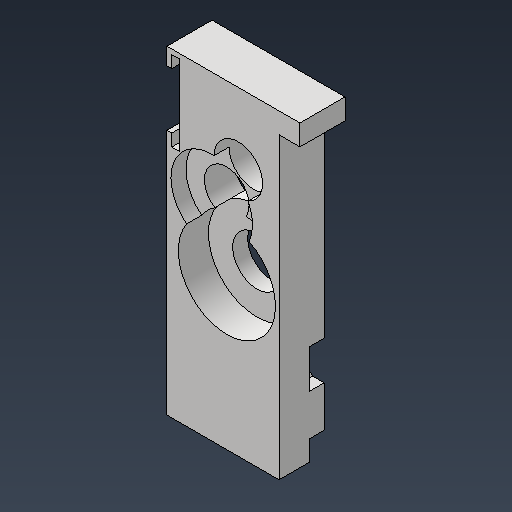
# Autodesk Inventor part: RightGearbox
Saved by Autodesk Inventor 2026.2 (Build 302298010, 298A)
## iProperties
Created: 2026-04-14
Part Number: RightGearbox
Material: Generic
Document SubType Name: Modeling
Designer: szymo
Density: 1 g/cm^3
Appearance: Default
Author: szymo
Autodesk Inventor part; units mm, degrees
ref_plane "YZ Plane" through (0, 0, 0) normal (1, 0, 0) x (0, 1, 0)
ref_plane "XZ Plane" through (0, 0, 0) normal (0, 1, 0) x (-1, 0, 0)
ref_plane "XY Plane" through (0, 0, 0) normal (0, 0, 1) x (1, 0, 0)
sketch "Sketch1" plane through (0, 0, 0) normal (0, 0, 1) x (1, 0, 0)
  circle A0 centre (14.7, -14.7) radius 5
  circle A1 centre (14.7, -14.7) radius 14.7 construction
  circle A2 centre (14.7, -55.6371) radius 5
  circle A3 centre (14.7, -55.6371) radius 14.7 construction
  line L0 (23.1, 0) -> (0, 0)
  line L1 (0, 0) -> (0, -65.8371)
  line L2 (0, -65.8371) -> (23.1, -65.8371)
  line L3 (23.1, -65.8371) -> (23.1, 0)
  circle A4 centre (12.35, -35.2722) radius 5
  line L4 (20.7104, -53.1622) -> (25.128, -48.7446)
  arc A5 (25.128, -48.7446) -> (21.5925, -45.2091) centre (14.7, -55.6371) ccw
  line L5 (21.5925, -45.2091) -> (17.1749, -49.6267)
  arc A6 (20.7104, -53.1622) -> (17.1749, -49.6267) centre (14.7, -55.6371) ccw construction
  arc A7 (4.272, -62.5296) -> (7.8075, -66.0651) centre (14.7, -55.6371) ccw
  line L6 (4.272, -62.5296) -> (8.6896, -58.1119)
  line L7 (12.2251, -61.6475) -> (7.8075, -66.0651)
  line L8 (20.7104, -53.1622) -> (23.1, -53.1622)
  line L9 (21.5925, -45.2091) -> (23.1, -45.2091)
  line L10 (12.2251, -61.6475) -> (8.6896, -58.1119)
  line L11 (20.7104, -53.1622) -> (17.1749, -49.6267)
  line L12 (12.2251, -61.6475) -> (23.1, -61.6475)
  circle A8 centre (9.2226, -23.0665) radius 4.2 construction
  circle A9 centre (9.2226, -23.0665) radius 8 construction
  circle A10 centre (12.35, -35.2722) radius 9.6 construction
  circle A11 centre (12.35, -35.2722) radius 10
  circle A12 centre (9.2226, -23.0665) radius 4.6
  circle A13 centre (9.2226, -23.0665) radius 8.4
  arc A14 (8.6896, -58.1119) -> (12.2251, -61.6475) centre (14.7, -55.6371) ccw construction
  line L13 (2.5, -1) -> (1.5, -1)
  line L14 (1.5, -1) -> (1.5, -17)
  line L15 (1.5, -17) -> (2.5, -17)
  line L16 (2.5, -17) -> (2.5, -1)
  line L17 (1.5, -1) -> (1, -1)
  line L18 (1, -1) -> (1, -3.5)
  line L19 (1, -3.5) -> (0, -3.5)
  line L20 (2.5, -17) -> (2.5, -17.5)
  line L21 (2.5, -17.5) -> (1, -17.5)
  line L22 (1, -17.5) -> (1, -15)
  line L23 (1, -15) -> (0, -15)
  line L24 (23.1, 0) -> (27.4, 0)
  line L25 (27.4, 0) -> (27.4, -4.272)
  line L26 (27.4, -4.272) -> (23.1, -4.272)
  line L27 (7.8075, -4.272) -> (12.2251, -8.6896)
  arc A15 (12.2251, -8.6896) -> (8.6896, -12.2251) centre (14.7, -14.7) ccw
  line L28 (8.6896, -12.2251) -> (4.272, -7.8075)
  arc A16 (7.8075, -4.272) -> (4.272, -7.8075) centre (14.7, -14.7) ccw
  line L29 (7.8075, -4.272) -> (23.1, -4.272)
  circle A17 centre (14.7, -14.7) radius 14.7 construction
  circle A18 centre (14.7, -14.7) radius 14 construction
  circle A19 centre (14.7, -14.7) radius 5 projected
  circle A20 centre (14.7, -14.7) radius 14 construction
  line L30 (10.5645, -8.4432) -> (7.6984, -5.5771) construction
  arc A21 (10.5645, -8.4432) -> (8.4432, -10.5645) centre (14.7, -14.7) ccw construction
  line L31 (5.5771, -7.6984) -> (8.4432, -10.5645) construction
  arc A22 (7.6984, -5.5771) -> (5.5771, -7.6984) centre (14.7, -14.7) ccw construction
  circle A23 centre (14.7, -55.6371) radius 14.7 construction
  circle A24 centre (14.7, -55.6371) radius 14 construction
  line L32 (18.8355, -49.3803) -> (21.7016, -46.5142) projected
  arc A25 (23.8229, -48.6355) -> (21.7016, -46.5142) centre (14.7, -55.6371) ccw projected
  line L33 (23.8229, -48.6355) -> (20.9568, -51.5016) projected
  arc A26 (20.9568, -51.5016) -> (18.8355, -49.3803) centre (14.7, -55.6371) ccw projected
  arc A27 (5.5771, -62.6387) -> (7.6984, -64.76) centre (14.7, -55.6371) ccw projected
  line L34 (5.5771, -62.6387) -> (8.4432, -59.7726) projected
  arc A28 (8.4432, -59.7726) -> (10.5645, -61.8939) centre (14.7, -55.6371) ccw projected
  line L35 (10.5645, -61.8939) -> (7.6984, -64.76) projected
  circle A29 centre (14.7, -55.6371) radius 5 projected
  circle A30 centre (14.7, -55.6371) radius 14 construction
  arc A31 (15.7399, -27.7508) -> (15.8311, -26.3256) centre (9.8372, -26.6574) ccw projected
  arc A32 (15.8311, -26.3256) -> (15.3581, -26.1557) centre (12.35, -35.2722) ccw projected
  arc A33 (15.3581, -26.1557) -> (14.5215, -27.3131) centre (19.7705, -30.2259) ccw projected
  arc A34 (14.5215, -27.3131) -> (14.102, -27.2104) centre (12.35, -35.2722) ccw projected
  arc A35 (14.102, -27.2104) -> (13.8949, -25.7973) centre (8.101, -27.3681) ccw projected
  arc A36 (13.8949, -25.7973) -> (13.3969, -25.7295) centre (12.35, -35.2722) ccw projected
  arc A37 (13.3969, -25.7295) -> (12.8193, -27.0356) centre (18.5592, -28.7934) ccw projected
  arc A38 (12.8193, -27.0356) -> (12.3876, -27.0223) centre (12.35, -35.2722) ccw projected
  arc A39 (12.3876, -27.0223) -> (11.8912, -25.6832) centre (6.5505, -28.4242) ccw projected
  arc A40 (11.8912, -25.6832) -> (11.39, -25.7203) centre (12.35, -35.2722) ccw projected
  arc A41 (11.39, -25.7203) -> (11.0965, -27.118) centre (17.0765, -27.644) ccw projected
  arc A42 (11.0965, -27.118) -> (10.6715, -27.1948) centre (12.35, -35.2722) ccw projected
  arc A43 (10.6715, -27.1948) -> (9.9076, -25.9881) centre (5.2535, -29.7796) ccw projected
  arc A44 (9.9076, -25.9881) -> (9.425, -26.1287) centre (12.35, -35.2722) ccw projected
  arc A45 (9.425, -26.1287) -> (9.4286, -27.5568) centre (15.3872, -26.828) ccw projected
  arc A46 (9.4286, -27.5568) -> (9.0288, -27.7203) centre (12.35, -35.2722) ccw projected
  arc A47 (9.0288, -27.7203) -> (8.0307, -26.6988) centre (4.2666, -31.3751) ccw projected
  arc A48 (8.0307, -26.6988) -> (7.5879, -26.9366) centre (12.35, -35.2722) ccw projected
  arc A49 (7.5879, -26.9366) -> (7.8883, -28.3328) centre (13.5652, -26.3811) ccw projected
  arc A50 (7.8883, -28.3328) -> (7.5312, -28.5758) centre (12.35, -35.2722) ccw projected
  arc A51 (7.5312, -28.5758) -> (6.3426, -27.7842) centre (3.633, -33.1409) ccw projected
  arc A52 (6.3426, -27.7842) -> (5.9589, -28.1088) centre (12.35, -35.2722) ccw projected
  arc A53 (5.9589, -28.1088) -> (6.543, -29.4121) centre (11.6901, -26.3227) ccw projected
  arc A54 (6.543, -29.4121) -> (6.2443, -29.724) centre (12.35, -35.2722) ccw projected
  arc A55 (6.2443, -29.724) -> (4.917, -29.1968) centre (3.3803, -34.9999) ccw projected
  arc A56 (4.917, -29.1968) -> (4.6092, -29.5942) centre (12.35, -35.2722) ccw projected
  arc A57 (4.6092, -29.5942) -> (5.4515, -30.7475) centre (9.8438, -26.6555) ccw projected
  arc A58 (5.4515, -30.7475) -> (5.2242, -31.1147) centre (12.35, -35.2722) ccw projected
  arc A59 (5.2242, -31.1147) -> (3.8163, -30.875) centre (3.5197, -36.8707) ccw projected
  arc A60 (3.8163, -30.875) -> (3.5978, -31.3276) centre (12.35, -35.2722) ccw projected
  arc A61 (3.5978, -31.3276) -> (4.6615, -32.2806) centre (8.107, -27.3648) ccw projected
  arc A62 (4.6615, -32.2806) -> (4.5155, -32.6871) centre (12.35, -35.2722) ccw projected
  arc A63 (4.5155, -32.6871) -> (3.0885, -32.7453) centre (4.045, -38.6717) ccw projected
  arc A64 (3.0885, -32.7453) -> (2.969, -33.2335) centre (12.35, -35.2722) ccw projected
  arc A65 (2.969, -33.2335) -> (4.2075, -33.9445) centre (6.5557, -28.4198) ccw projected
  arc A66 (4.2075, -33.9445) -> (4.1492, -34.3725) centre (12.35, -35.2722) ccw projected
  arc A67 (4.1492, -34.3725) -> (2.7655, -34.7261) centre (4.9333, -40.3241) ccw projected
  arc A68 (2.7655, -34.7261) -> (2.7501, -35.2285) centre (12.35, -35.2722) ccw projected
  arc A69 (2.7501, -35.2285) -> (4.1094, -35.6665) centre (5.2576, -29.7742) ccw projected
  arc A70 (4.1094, -35.6665) -> (4.1414, -36.0972) centre (12.35, -35.2722) ccw projected
  arc A71 (4.1414, -36.0972) -> (2.8615, -36.7308) centre (6.1457, -41.7557) ccw projected
  arc A72 (2.8615, -36.7308) -> (2.9508, -37.2254) centre (12.35, -35.2722) ccw projected
  arc A73 (2.9508, -37.2254) -> (4.3715, -37.3712) centre (4.2695, -31.369) ccw projected
  arc A74 (4.3715, -37.3712) -> (4.4923, -37.7858) centre (12.35, -35.2722) ccw projected
  arc A75 (4.4923, -37.7858) -> (3.3721, -38.6717) centre (7.6293, -42.904) ccw projected
  arc A76 (3.3721, -38.6717) -> (3.5623, -39.1369) centre (12.35, -35.2722) ccw projected
  arc A77 (3.5623, -39.1369) -> (4.9822, -38.9841) centre (3.6346, -33.1343) ccw projected
  arc A78 (4.9822, -38.9841) -> (5.1866, -39.3646) centre (12.35, -35.2722) ccw projected
  arc A79 (5.1866, -39.3646) -> (4.275, -40.464) centre (9.3192, -43.7187) ccw projected
  arc A80 (4.275, -40.464) -> (4.5578, -40.8795) centre (12.35, -35.2722) ccw projected
  arc A81 (4.5578, -40.8795) -> (5.915, -40.4349) centre (3.3805, -34.993) ccw projected
  arc A82 (5.915, -40.4349) -> (6.194, -40.7646) centre (12.35, -35.2722) ccw projected
  arc A83 (6.194, -40.7646) -> (5.5309, -42.0295) centre (11.1416, -44.1643) ccw projected
  arc A84 (5.5309, -42.0295) -> (5.8939, -42.3771) centre (12.35, -35.2722) ccw projected
  arc A85 (5.8939, -42.3771) -> (7.129, -41.66) centre (3.5185, -36.864) ccw projected
  arc A86 (7.129, -41.66) -> (7.4704, -41.9244) centre (12.35, -35.2722) ccw projected
  arc A87 (7.4704, -41.9244) -> (7.0849, -43.2996) centre (13.0167, -44.2212) ccw projected
  arc A88 (7.0849, -43.2996) -> (7.5122, -43.5641) centre (12.35, -35.2722) ccw projected
  arc A89 (7.5122, -43.5641) -> (8.5711, -42.6059) centre (4.0424, -38.6654) ccw projected
  arc A90 (8.5711, -42.6059) -> (8.9601, -42.7936) centre (12.35, -35.2722) ccw projected
  arc A91 (8.9601, -42.7936) -> (8.8689, -44.2188) centre (14.8628, -43.887) ccw projected
  arc A92 (8.8689, -44.2188) -> (9.3419, -44.3887) centre (12.35, -35.2722) ccw projected
  arc A93 (9.3419, -44.3887) -> (10.1785, -43.2313) centre (4.9295, -40.3185) ccw projected
  arc A94 (10.1785, -43.2313) -> (10.598, -43.334) centre (12.35, -35.2722) ccw projected
  arc A95 (10.598, -43.334) -> (10.8051, -44.7471) centre (16.599, -43.1764) ccw projected
  arc A96 (10.8051, -44.7471) -> (11.3031, -44.815) centre (12.35, -35.2722) ccw projected
  arc A97 (11.3031, -44.815) -> (11.8807, -43.5089) centre (6.1408, -41.751) ccw projected
  arc A98 (11.8807, -43.5089) -> (12.3124, -43.5221) centre (12.35, -35.2722) ccw projected
  arc A99 (12.3124, -43.5221) -> (12.8088, -44.8612) centre (18.1495, -42.1202) ccw projected
  arc A100 (12.8088, -44.8612) -> (13.31, -44.8241) centre (12.35, -35.2722) ccw projected
  arc A101 (13.31, -44.8241) -> (13.6035, -43.4264) centre (7.6235, -42.9004) ccw projected
  arc A102 (13.6035, -43.4264) -> (14.0285, -43.3497) centre (12.35, -35.2722) ccw projected
  arc A103 (14.0285, -43.3497) -> (14.7924, -44.5563) centre (19.4465, -40.7648) ccw projected
  arc A104 (14.7924, -44.5563) -> (15.275, -44.4158) centre (12.35, -35.2722) ccw projected
  arc A105 (15.275, -44.4158) -> (15.2714, -42.9876) centre (9.3128, -43.7164) ccw projected
  arc A106 (15.2714, -42.9876) -> (15.6712, -42.8242) centre (12.35, -35.2722) ccw projected
  arc A107 (15.6712, -42.8242) -> (16.6693, -43.8456) centre (20.4334, -39.1693) ccw projected
  arc A108 (16.6693, -43.8456) -> (17.1121, -43.6078) centre (12.35, -35.2722) ccw projected
  arc A109 (17.1121, -43.6078) -> (16.8117, -42.2116) centre (11.1348, -44.1634) ccw projected
  arc A110 (16.8117, -42.2116) -> (17.1688, -41.9686) centre (12.35, -35.2722) ccw projected
  arc A111 (17.1688, -41.9686) -> (18.3574, -42.7603) centre (21.067, -37.4035) ccw projected
  arc A112 (18.3574, -42.7603) -> (18.7411, -42.4356) centre (12.35, -35.2722) ccw projected
  arc A113 (18.7411, -42.4356) -> (18.157, -41.1324) centre (13.0099, -44.2217) ccw projected
  arc A114 (18.157, -41.1324) -> (18.4557, -40.8204) centre (12.35, -35.2722) ccw projected
  arc A115 (18.4557, -40.8204) -> (19.783, -41.3476) centre (21.3197, -35.5446) ccw projected
  arc A116 (19.783, -41.3476) -> (20.0908, -40.9503) centre (12.35, -35.2722) ccw projected
  arc A117 (20.0908, -40.9503) -> (19.2485, -39.7969) centre (14.8562, -43.8889) ccw projected
  arc A118 (19.2485, -39.7969) -> (19.4758, -39.4297) centre (12.35, -35.2722) ccw projected
  arc A119 (19.4758, -39.4297) -> (20.8837, -39.6694) centre (21.1803, -33.6737) ccw projected
  arc A120 (20.8837, -39.6694) -> (21.1022, -39.2168) centre (12.35, -35.2722) ccw projected
  arc A121 (21.1022, -39.2168) -> (20.0385, -38.2638) centre (16.593, -43.1796) ccw projected
  arc A122 (20.0385, -38.2638) -> (20.1845, -37.8573) centre (12.35, -35.2722) ccw projected
  arc A123 (20.1845, -37.8573) -> (21.6115, -37.7991) centre (20.655, -31.8727) ccw projected
  arc A124 (21.6115, -37.7991) -> (21.731, -37.3109) centre (12.35, -35.2722) ccw projected
  arc A125 (21.731, -37.3109) -> (20.4925, -36.5999) centre (18.1443, -42.1246) ccw projected
  arc A126 (20.4925, -36.5999) -> (20.5508, -36.1719) centre (12.35, -35.2722) ccw projected
  arc A127 (20.5508, -36.1719) -> (21.9345, -35.8183) centre (19.7667, -30.2203) ccw projected
  arc A128 (21.9345, -35.8183) -> (21.9499, -35.3159) centre (12.35, -35.2722) ccw projected
  arc A129 (21.9499, -35.3159) -> (20.5906, -34.878) centre (19.4424, -40.7702) ccw projected
  arc A130 (20.5906, -34.878) -> (20.5586, -34.4472) centre (12.35, -35.2722) ccw projected
  arc A131 (20.5586, -34.4472) -> (21.8385, -33.8136) centre (18.5543, -28.7887) ccw projected
  arc A132 (21.8385, -33.8136) -> (21.7492, -33.319) centre (12.35, -35.2722) ccw projected
  arc A133 (21.7492, -33.319) -> (20.3285, -33.1733) centre (20.4305, -39.1755) ccw projected
  arc A134 (20.3285, -33.1733) -> (20.2077, -32.7586) centre (12.35, -35.2722) ccw projected
  arc A135 (20.2077, -32.7586) -> (21.3279, -31.8727) centre (17.0707, -27.6404) ccw projected
  arc A136 (21.3279, -31.8727) -> (21.1377, -31.4075) centre (12.35, -35.2722) ccw projected
  arc A137 (21.1377, -31.4075) -> (19.7178, -31.5603) centre (21.0654, -37.4101) ccw projected
  arc A138 (19.7178, -31.5603) -> (19.5134, -31.1798) centre (12.35, -35.2722) ccw projected
  arc A139 (19.5134, -31.1798) -> (20.425, -30.0804) centre (15.3808, -26.8257) ccw projected
  arc A140 (20.425, -30.0804) -> (20.1422, -29.6649) centre (12.35, -35.2722) ccw projected
  arc A141 (20.1422, -29.6649) -> (18.785, -30.1096) centre (21.3195, -35.5514) ccw projected
  arc A142 (18.785, -30.1096) -> (18.506, -29.7799) centre (12.35, -35.2722) ccw projected
  arc A143 (18.506, -29.7799) -> (19.1691, -28.515) centre (13.5584, -26.3801) ccw projected
  arc A144 (19.1691, -28.515) -> (18.8061, -28.1674) centre (12.35, -35.2722) ccw projected
  arc A145 (18.8061, -28.1674) -> (17.571, -28.8845) centre (21.1815, -33.6804) ccw projected
  arc A146 (17.571, -28.8845) -> (17.2296, -28.62) centre (12.35, -35.2722) ccw projected
  arc A147 (17.2296, -28.62) -> (17.6151, -27.2449) centre (11.6833, -26.3232) ccw projected
  arc A148 (17.6151, -27.2449) -> (17.1878, -26.9803) centre (12.35, -35.2722) ccw projected
  arc A149 (17.1878, -26.9803) -> (16.1289, -27.9385) centre (20.6576, -31.879) ccw projected
  arc A150 (16.1289, -27.9385) -> (15.7399, -27.7508) centre (12.35, -35.2722) ccw projected
  circle A151 centre (9.2226, -23.0665) radius 1.25 projected
  arc A152 (17.1791, -22.2335) -> (16.0134, -21.9938) centre (15.5957, -26.9788) ccw projected
  arc A153 (16.0134, -21.9938) -> (15.948, -21.6398) centre (9.2226, -23.0665) ccw projected
  arc A154 (15.948, -21.6398) -> (16.9509, -20.9991) centre (13.7752, -17.1338) ccw projected
  arc A155 (16.9509, -20.9991) -> (16.8321, -20.5974) centre (9.2226, -23.0665) ccw projected
  arc A156 (16.8321, -20.5974) -> (15.642, -20.6053) centre (16.2699, -25.5683) ccw projected
  arc A157 (15.642, -20.6053) -> (15.5044, -20.2727) centre (9.2226, -23.0665) ccw projected
  arc A158 (15.5044, -20.2727) -> (16.3521, -19.4375) centre (12.4422, -16.3169) ccw projected
  arc A159 (16.3521, -19.4375) -> (16.1524, -19.0693) centre (9.2226, -23.0665) ccw projected
  arc A160 (16.1524, -19.0693) -> (14.99, -19.3244) centre (16.636, -24.0484) ccw projected
  arc A161 (14.99, -19.3244) -> (14.7862, -19.0277) centre (9.2226, -23.0665) ccw projected
  arc A162 (14.7862, -19.0277) -> (15.4418, -18.0345) centre (10.9685, -15.795) ccw projected
  arc A163 (15.4418, -18.0345) -> (15.1699, -17.7159) centre (9.2226, -23.0665) ccw projected
  arc A164 (15.1699, -17.7159) -> (14.0859, -18.2071) centre (16.6782, -22.4856) ccw projected
  arc A165 (14.0859, -18.2071) -> (13.825, -17.9592) centre (9.2226, -23.0665) ccw projected
  arc A166 (13.825, -17.9592) -> (14.2597, -16.8514) centre (9.4186, -15.5909) ccw projected
  arc A167 (14.2597, -16.8514) -> (13.9275, -16.5963) centre (9.2226, -23.0665) ccw projected
  arc A168 (13.9275, -16.5963) -> (12.9693, -17.3022) centre (16.3945, -20.9482) ccw projected
  arc A169 (12.9693, -17.3022) -> (12.6625, -17.114) centre (9.2226, -23.0665) ccw projected
  arc A170 (12.6625, -17.114) -> (12.8574, -15.9399) centre (7.86, -15.7135) ccw projected
  arc A171 (12.8574, -15.9399) -> (12.4795, -15.7595) centre (9.2226, -23.0665) ccw projected
  arc A172 (12.4795, -15.7595) -> (11.689, -16.6491) centre (15.7974, -19.5034) ccw projected
  arc A173 (11.689, -16.6491) -> (11.3498, -16.5288) centre (9.2226, -23.0665) ccw projected
  arc A174 (11.3498, -16.5288) -> (11.2963, -15.3399) centre (6.361, -16.1575) ccw projected
  arc A175 (11.2963, -15.3399) -> (10.8891, -15.242) centre (9.2226, -23.0665) ccw projected
  arc A176 (10.8891, -15.242) -> (10.3009, -16.2766) centre (14.9129, -18.2143) ccw projected
  arc A177 (10.3009, -16.2766) -> (9.944, -16.2295) centre (9.2226, -23.0665) ccw projected
  arc A178 (9.944, -16.2295) -> (9.6445, -15.0776) centre (4.9871, -16.9034) ccw projected
  arc A179 (9.6445, -15.0776) -> (9.2259, -15.0665) centre (9.2226, -23.0665) ccw projected
  arc A180 (9.2259, -15.0665) -> (8.8656, -16.2008) centre (13.7797, -17.1372) ccw projected
  arc A181 (8.8656, -16.2008) -> (8.5068, -16.2289) centre (9.2226, -23.0665) ccw projected
  arc A182 (8.5068, -16.2289) -> (7.9743, -15.1645) centre (3.7983, -17.9187) ccw projected
  arc A183 (7.9743, -15.1645) -> (7.5625, -15.2406) centre (9.2226, -23.0665) ccw projected
  arc A184 (7.5625, -15.2406) -> (7.4459, -16.425) centre (12.4474, -16.3193) ccw projected
  arc A185 (7.4459, -16.425) -> (7.1008, -16.5271) centre (9.2226, -23.0665) ccw projected
  arc A186 (7.1008, -16.5271) -> (6.3587, -15.5967) centre (2.8465, -19.159) ccw projected
  arc A187 (6.3587, -15.5967) -> (5.9717, -15.7568) centre (9.2226, -23.0665) ccw projected
  arc A188 (5.9717, -15.7568) -> (6.1039, -16.9396) centre (10.9741, -15.7963) ccw projected
  arc A189 (6.1039, -16.9396) -> (5.7875, -17.1112) centre (9.2226, -23.0665) ccw projected
  arc A190 (5.7875, -17.1112) -> (4.8682, -16.3554) centre (2.1734, -20.5701) ccw projected
  arc A191 (4.8682, -16.3554) -> (4.523, -16.5925) centre (9.2226, -23.0665) ccw projected
  arc A192 (4.523, -16.5925) -> (4.8982, -17.7219) centre (9.4242, -15.591) ccw projected
  arc A193 (4.8982, -17.7219) -> (4.6244, -17.9555) centre (9.2226, -23.0665) ccw projected
  arc A194 (4.6244, -17.9555) -> (3.5681, -17.4074) centre (1.8085, -22.0902) ccw projected
  arc A195 (3.5681, -17.4074) -> (3.2796, -17.711) centre (9.2226, -23.0665) ccw projected
  arc A196 (3.2796, -17.711) -> (3.8815, -18.7378) centre (7.8656, -15.7125) ccw projected
  arc A197 (3.8815, -18.7378) -> (3.6623, -19.0232) centre (9.2226, -23.0665) ccw projected
  arc A198 (3.6623, -19.0232) -> (2.515, -18.7067) centre (1.7675, -23.653) ccw projected
  arc A199 (2.515, -18.7067) -> (2.296, -19.0637) centre (9.2226, -23.0665) ccw projected
  arc A200 (2.296, -19.0637) -> (3.0982, -19.9428) centre (6.3663, -16.1553) ccw projected
  arc A201 (3.0982, -19.9428) -> (2.9431, -20.2676) centre (9.2226, -23.0665) ccw projected
  arc A202 (2.9431, -20.2676) -> (1.7551, -20.1965) centre (2.0523, -25.1902) ccw projected
  arc A203 (1.7551, -20.1965) -> (1.6152, -20.5913) centre (9.2226, -23.0665) ccw projected
  arc A204 (1.6152, -20.5913) -> (2.5826, -21.2844) centre (4.9918, -16.9002) ccw projected
  arc A205 (2.5826, -21.2844) -> (2.4984, -21.6344) centre (9.2226, -23.0665) ccw projected
  arc A206 (2.4984, -21.6344) -> (1.3216, -21.8118) centre (2.6506, -26.6346) ccw projected
  arc A207 (1.3216, -21.8118) -> (1.2668, -22.227) centre (9.2226, -23.0665) ccw projected
  arc A208 (1.2668, -22.227) -> (2.3572, -22.7039) centre (3.8022, -17.9146) ccw projected
  arc A209 (2.3572, -22.7039) -> (2.3476, -23.0637) centre (9.2226, -23.0665) ccw projected
  arc A210 (2.3476, -23.0637) -> (1.2334, -23.4819) centre (3.536, -27.923) ccw projected
  arc A211 (1.2334, -23.4819) -> (1.2661, -23.8995) centre (9.2226, -23.0665) ccw projected
  arc A212 (1.2661, -23.8995) -> (2.4318, -24.1392) centre (2.8495, -19.1542) ccw projected
  arc A213 (2.4318, -24.1392) -> (2.4973, -24.4932) centre (9.2226, -23.0665) ccw projected
  arc A214 (2.4973, -24.4932) -> (1.4944, -25.1339) centre (4.67, -28.9992) ccw projected
  arc A215 (1.4944, -25.1339) -> (1.6132, -25.5355) centre (9.2226, -23.0665) ccw projected
  arc A216 (1.6132, -25.5355) -> (2.8033, -25.5277) centre (2.1753, -20.5647) ccw projected
  arc A217 (2.8033, -25.5277) -> (2.9409, -25.8603) centre (9.2226, -23.0665) ccw projected
  arc A218 (2.9409, -25.8603) -> (2.0931, -26.6955) centre (6.003, -29.8161) ccw projected
  arc A219 (2.0931, -26.6955) -> (2.2928, -27.0637) centre (9.2226, -23.0665) ccw projected
  arc A220 (2.2928, -27.0637) -> (3.4552, -26.8086) centre (1.8092, -22.0846) ccw projected
  arc A221 (3.4552, -26.8086) -> (3.659, -27.1053) centre (9.2226, -23.0665) ccw projected
  arc A222 (3.659, -27.1053) -> (3.0034, -28.0985) centre (7.4767, -30.338) ccw projected
  arc A223 (3.0034, -28.0985) -> (3.2753, -28.4171) centre (9.2226, -23.0665) ccw projected
  arc A224 (3.2753, -28.4171) -> (4.3593, -27.9259) centre (1.767, -23.6474) ccw projected
  arc A225 (4.3593, -27.9259) -> (4.6203, -28.1738) centre (9.2226, -23.0665) ccw projected
  arc A226 (4.6203, -28.1738) -> (4.1855, -29.2816) centre (9.0267, -30.5421) ccw projected
  arc A227 (4.1855, -29.2816) -> (4.5177, -29.5367) centre (9.2226, -23.0665) ccw projected
  arc A228 (4.5177, -29.5367) -> (5.4759, -28.8308) centre (2.0507, -25.1848) ccw projected
  arc A229 (5.4759, -28.8308) -> (5.7827, -29.019) centre (9.2226, -23.0665) ccw projected
  arc A230 (5.7827, -29.019) -> (5.5878, -30.1931) centre (10.5852, -30.4195) ccw projected
  arc A231 (5.5878, -30.1931) -> (5.9658, -30.3735) centre (9.2226, -23.0665) ccw projected
  arc A232 (5.9658, -30.3735) -> (6.7562, -29.4839) centre (2.6479, -26.6296) ccw projected
  arc A233 (6.7562, -29.4839) -> (7.0955, -29.6041) centre (9.2226, -23.0665) ccw projected
  arc A234 (7.0955, -29.6041) -> (7.1489, -30.7931) centre (12.0842, -29.9755) ccw projected
  arc A235 (7.1489, -30.7931) -> (7.5562, -30.891) centre (9.2226, -23.0665) ccw projected
  arc A236 (7.5562, -30.891) -> (8.1444, -29.8564) centre (3.5324, -27.9187) ccw projected
  arc A237 (8.1444, -29.8564) -> (8.5012, -29.9035) centre (9.2226, -23.0665) ccw projected
  arc A238 (8.5012, -29.9035) -> (8.8007, -31.0554) centre (13.4581, -29.2296) ccw projected
  arc A239 (8.8007, -31.0554) -> (9.2194, -31.0665) centre (9.2226, -23.0665) ccw projected
  arc A240 (9.2194, -31.0665) -> (9.5796, -29.9322) centre (4.6655, -28.9958) ccw projected
  arc A241 (9.5796, -29.9322) -> (9.9385, -29.9041) centre (9.2226, -23.0665) ccw projected
  arc A242 (9.9385, -29.9041) -> (10.4709, -30.9685) centre (14.647, -28.2143) ccw projected
  arc A243 (10.4709, -30.9685) -> (10.8827, -30.8924) centre (9.2226, -23.0665) ccw projected
  arc A244 (10.8827, -30.8924) -> (10.9993, -29.708) centre (5.9979, -29.8137) ccw projected
  arc A245 (10.9993, -29.708) -> (11.3445, -29.6059) centre (9.2226, -23.0665) ccw projected
  arc A246 (11.3445, -29.6059) -> (12.0865, -30.5363) centre (15.5987, -26.974) ccw projected
  arc A247 (12.0865, -30.5363) -> (12.4735, -30.3762) centre (9.2226, -23.0665) ccw projected
  arc A248 (12.4735, -30.3762) -> (12.3413, -29.1934) centre (7.4712, -30.3367) ccw projected
  arc A249 (12.3413, -29.1934) -> (12.6577, -29.0218) centre (9.2226, -23.0665) ccw projected
  arc A250 (12.6577, -29.0218) -> (13.577, -29.7776) centre (16.2718, -25.5629) ccw projected
  arc A251 (13.577, -29.7776) -> (13.9223, -29.5405) centre (9.2226, -23.0665) ccw projected
  arc A252 (13.9223, -29.5405) -> (13.547, -28.4111) centre (9.021, -30.5419) ccw projected
  arc A253 (13.547, -28.4111) -> (13.8208, -28.1775) centre (9.2226, -23.0665) ccw projected
  arc A254 (13.8208, -28.1775) -> (14.8772, -28.7256) centre (16.6368, -24.0428) ccw projected
  arc A255 (14.8772, -28.7256) -> (15.1656, -28.422) centre (9.2226, -23.0665) ccw projected
  arc A256 (15.1656, -28.422) -> (14.5637, -27.3952) centre (10.5796, -30.4205) ccw projected
  arc A257 (14.5637, -27.3952) -> (14.783, -27.1098) centre (9.2226, -23.0665) ccw projected
  arc A258 (14.783, -27.1098) -> (15.9302, -27.4263) centre (16.6777, -22.48) ccw projected
  arc A259 (15.9302, -27.4263) -> (16.1492, -27.0693) centre (9.2226, -23.0665) ccw projected
  arc A260 (16.1492, -27.0693) -> (15.347, -26.1902) centre (12.079, -29.9777) ccw projected
  arc A261 (15.347, -26.1902) -> (15.5021, -25.8654) centre (9.2226, -23.0665) ccw projected
  arc A262 (15.5021, -25.8654) -> (16.6901, -25.9365) centre (16.3929, -20.9428) ccw projected
  arc A263 (16.6901, -25.9365) -> (16.8301, -25.5417) centre (9.2226, -23.0665) ccw projected
  arc A264 (16.8301, -25.5417) -> (15.8626, -24.8486) centre (13.4535, -29.2328) ccw projected
  arc A265 (15.8626, -24.8486) -> (15.9468, -24.4986) centre (9.2226, -23.0665) ccw projected
  arc A266 (15.9468, -24.4986) -> (17.1236, -24.3212) centre (15.7947, -19.4984) ccw projected
  arc A267 (17.1236, -24.3212) -> (17.1785, -23.906) centre (9.2226, -23.0665) ccw projected
  arc A268 (17.1785, -23.906) -> (16.088, -23.4291) centre (14.643, -28.2184) ccw projected
  arc A269 (16.088, -23.4291) -> (16.0976, -23.0693) centre (9.2226, -23.0665) ccw projected
  arc A270 (16.0976, -23.0693) -> (17.2118, -22.651) centre (14.9092, -18.21) ccw projected
  arc A271 (17.2118, -22.651) -> (17.1791, -22.2335) centre (9.2226, -23.0665) ccw projected
  circle A272 centre (9.2226, -23.0665) radius 1.25 projected
  arc A273 (5.455, -24.9226) -> (6.8523, -24.6489) centre (5.4549, -21.218) ccw projected
  arc A274 (6.8523, -24.6489) -> (7.0791, -24.9448) centre (9.2226, -23.0665) ccw projected
  arc A275 (7.0791, -24.9448) -> (6.4521, -26.2231) centre (10.0296, -27.1849) ccw projected
  arc A276 (6.4521, -26.2231) -> (6.8878, -26.5577) centre (9.2226, -23.0665) ccw projected
  arc A277 (6.8878, -26.5577) -> (7.9611, -25.6221) centre (5.0354, -23.3495) ccw projected
  arc A278 (7.9611, -25.6221) -> (8.3054, -25.7649) centre (9.2226, -23.0665) ccw projected
  arc A279 (8.3054, -25.7649) -> (8.4016, -27.1855) centre (11.9807, -26.2297) ccw projected
  arc A280 (8.4016, -27.1855) -> (8.9462, -27.2574) centre (9.2226, -23.0665) ccw projected
  arc A281 (8.9462, -27.2574) -> (9.4079, -25.9105) centre (5.7379, -25.4052) ccw projected
  arc A282 (9.4079, -25.9105) -> (9.7775, -25.862) centre (9.2226, -23.0665) ccw projected
  arc A283 (9.7775, -25.862) -> (10.5711, -27.0442) centre (13.1928, -24.4268) ccw projected
  arc A284 (10.5711, -27.0442) -> (11.0787, -26.8341) centre (9.2226, -23.0665) ccw projected
  arc A285 (11.0787, -26.8341) -> (10.805, -25.4368) centre (7.3742, -26.8342) ccw projected
  arc A286 (10.805, -25.4368) -> (11.1009, -25.21) centre (9.2226, -23.0665) ccw projected
  arc A287 (11.1009, -25.21) -> (12.3792, -25.837) centre (13.3411, -22.2595) ccw projected
  arc A288 (12.3792, -25.837) -> (12.7138, -25.4013) centre (9.2226, -23.0665) ccw projected
  arc A289 (12.7138, -25.4013) -> (11.7782, -24.3281) centre (9.5057, -27.2537) ccw projected
  arc A290 (11.7782, -24.3281) -> (11.921, -23.9837) centre (9.2226, -23.0665) ccw projected
  arc A291 (11.921, -23.9837) -> (13.3416, -23.8875) centre (12.3858, -20.3084) ccw projected
  arc A292 (13.3416, -23.8875) -> (13.4135, -23.3429) centre (9.2226, -23.0665) ccw projected
  arc A293 (13.4135, -23.3429) -> (12.0666, -22.8813) centre (11.5613, -26.5512) ccw projected
  arc A294 (12.0666, -22.8813) -> (12.0181, -22.5116) centre (9.2226, -23.0665) ccw projected
  arc A295 (12.0181, -22.5116) -> (13.2003, -21.7181) centre (10.583, -19.0963) ccw projected
  arc A296 (13.2003, -21.7181) -> (12.9902, -21.2104) centre (9.2226, -23.0665) ccw projected
  arc A297 (12.9902, -21.2104) -> (11.5929, -21.4841) centre (12.9904, -24.915) ccw projected
  arc A298 (11.5929, -21.4841) -> (11.3661, -21.1882) centre (9.2226, -23.0665) ccw projected
  arc A299 (11.3661, -21.1882) -> (11.9932, -19.9099) centre (8.4156, -18.9481) ccw projected
  arc A300 (11.9932, -19.9099) -> (11.5574, -19.5753) centre (9.2226, -23.0665) ccw projected
  arc A301 (11.5574, -19.5753) -> (10.4842, -20.5109) centre (13.4098, -22.7834) ccw projected
  arc A302 (10.4842, -20.5109) -> (10.1398, -20.3681) centre (9.2226, -23.0665) ccw projected
  arc A303 (10.1398, -20.3681) -> (10.0437, -18.9475) centre (6.4645, -19.9033) ccw projected
  arc A304 (10.0437, -18.9475) -> (9.499, -18.8756) centre (9.2226, -23.0665) ccw projected
  arc A305 (9.499, -18.8756) -> (9.0374, -20.2225) centre (12.7073, -20.7278) ccw projected
  arc A306 (9.0374, -20.2225) -> (8.6677, -20.271) centre (9.2226, -23.0665) ccw projected
  arc A307 (8.6677, -20.271) -> (7.8742, -19.0888) centre (5.2525, -21.7061) ccw projected
  arc A308 (7.8742, -19.0888) -> (7.3665, -19.2989) centre (9.2226, -23.0665) ccw projected
  arc A309 (7.3665, -19.2989) -> (7.6402, -20.6962) centre (11.0711, -19.2988) ccw projected
  arc A310 (7.6402, -20.6962) -> (7.3444, -20.923) centre (9.2226, -23.0665) ccw projected
  arc A311 (7.3444, -20.923) -> (6.066, -20.296) centre (5.1042, -23.8735) ccw projected
  arc A312 (6.066, -20.296) -> (5.7314, -20.7317) centre (9.2226, -23.0665) ccw projected
  arc A313 (5.7314, -20.7317) -> (6.667, -21.8049) centre (8.9396, -18.8793) ccw projected
  arc A314 (6.667, -21.8049) -> (6.5242, -22.1493) centre (9.2226, -23.0665) ccw projected
  arc A315 (6.5242, -22.1493) -> (5.1037, -22.2454) centre (6.0594, -25.8246) ccw projected
  arc A316 (5.1037, -22.2454) -> (5.0317, -22.7901) centre (9.2226, -23.0665) ccw projected
  arc A317 (5.0317, -22.7901) -> (6.3786, -23.2517) centre (6.8839, -19.5818) ccw projected
  arc A318 (6.3786, -23.2517) -> (6.4272, -23.6214) centre (9.2226, -23.0665) ccw projected
  arc A319 (6.4272, -23.6214) -> (5.245, -24.4149) centre (7.8623, -27.0367) ccw projected
  arc A320 (5.245, -24.4149) -> (5.455, -24.9226) centre (9.2226, -23.0665) ccw projected
  line L36 (1.5, -17) -> (1.5, -1) projected
  line L37 (2.5, -17) -> (1.5, -17) projected
  line L38 (2.5, -1) -> (2.5, -17) projected
  line L39 (2.5, -1) -> (1.5, -1) projected
  point P0 (0, 0)
  point P1 (7.4744, -65.8371)
  point P2 (4.0542, -29.6883)
  point P3 (9.7, -14.6801)
  point P4 (16.7181, -19.2746)
  point P5 (16.9384, -26.387)
  point P6 (6.7821, -26.9657)
  point P7 (13.2375, -25.3117)
  point P8 (8.0355, -65.8371)
  dimension "d2" = 4.5
  dimension "d3" = 6.3
  dimension "d4" = 0.4
  dimension "d5" = 0.4
  dimension "d6" = 0.4
  dimension "d27" = 0
  dimension "d36" = 0.5
  dimension "d37" = 2.5
  dimension "d38" = 0.5
  dimension "d39" = 0.5
  dimension "d40" = 2.5
  dimension "d41" = 2
  dimension "d43" = 10
  dimension "d44" = 1
  dimension "d45" = 1
  dimension "d46" = 1
  dimension "d47" = 1
  dimension "d48" = 1
  dimension "d49" = 1
  dimension "d50" = 1
  dimension "d51" = 1
  dimension "d52" = 1
  dimension "d54" = 1
  dimension "d56" = 1
  dimension "d57" = 1
  constraints: 60 end point, 14 centre point, 13 coincident, 12 perpendicular, 12 point on circle, 7 parallel, 6 point on line, 6 tangent, 4 horizontal, 2 collinear, 1 vertical, 13 other
  measures "d2" distance edge to line of A3 L2
  measures "d3" distance edge to line of A1 L3
  measures "d27" distance from line of L6 A14.start
  measures "d36" distance between parallel lines of L14 L18
  measures "d37" distance between parallel lines of L19 L13
  measures "d38" distance between parallel lines of L22 L14
  measures "d39" distance between parallel lines of L21 L15
  measures "d40" distance between parallel lines of L21 L23
  measures "d41" distance edge to line of A1 L25
  measures "d43" diameter of A4
  measures "d44" distance between parallel lines of L28 L31
  measures "d45" distance between parallel lines of L27 L30
  measures "d46" radial gap between concentric circles of A22 A16
  measures "d47" radial gap between concentric circles of A15 A21
  measures "d48" distance between parallel lines of L33 L4
  measures "d49" distance between parallel lines of L5 L32
  measures "d50" radial gap between concentric circles of A5 A25
  measures "d51" radial gap between concentric circles of A6 A26
  measures "d52" radial gap between concentric circles of A28 A14
  measures "d54" radial gap between concentric circles of A7 A27
  measures "d56" distance between parallel lines of L6 L34
  measures "d57" distance between parallel lines of L7 L35
extrude "Extrusion5" add sketch "Sketch1" along normal blind 3.1 contours A0 A178 A179 A180 A181 A182 A183 A184 A185 A186 A187 A188 A189 A190 A191 A192 A193 A194 A195 A196 A197 A198 A199 A200 A201 A202 A203 A204 A205 A206 A207 A208 A209 A210 A211 A212 A213 A214 A215 A216 A217 A218 A219 A220 A221 A222 A223 A224 A225 A226 A227 A11 A13 | A13 A11 A262 A263 A264 A265 A266 A267 A268 A269 A270 A271 A152 A153 A154 A155 A156 A157 A158 A159 A0 | A0 A159 A158 A157 A156 A155 A154 A153 A152 A271 A270 A269 A268 A267 A266 A265 A264 A263 A262 A11 A12 A227 A226 A225 A224 A223 A222 A221 A220 A219 A218 A217 A216 A215 A214 A213 A212 A211 A210 A209 A208 A207 A206 A205 A204 A203 A202 A201 A200 A199 A198 A197 A196 A195 A194 A193 A192 A191 A190 A189 A188 A187 A186 A185 A184 A183 A182 A181 A180 A179 A178 | A13 A57 A58 A59 A60 A61 A62 A63 A64 A65 A66 A67 A68 A69 A70 A71 A72 A73 A74 A75 A76 A77 A78 A79 A80 A81 A82 A83 A84 A85 A86 A87 A88 A89 A90 A91 A92 A93 A94 A95 A96 A97 A98 A99 A100 A101 A102 A103 A104 A105 A106 A107 A108 A109 A110 A111 A112 A113 A114 A115 A116 A117 A118 A119 A120 A121 A122 A123 A124 A125 A126 A127 A128 A129 A130 A131 A132 A133 A134 A135 A136 A137 A138 A139 A140 A141 A142 A143 A144 A145 A146 A147 A148 A149 A150 A11 | A11 A227 A228 A56 A57 A13 | A11 A12 A49 A50 A51 A52 A53 A54 A55 A230 A229 A228 A56 A227 | A57 A56 A228 A55 A230 A231 A232 A233 A234 A235 A236 A237 A238 A239 A240 A241 A242 A4 A13 | A13 A4 A150 A149 A148 A147 A146 A145 A144 A143 A142 A141 A140 A139 A138 A137 A136 A135 A134 A133 A132 A131 A130 A129 A128 A127 A126 A125 A124 A123 A122 A121 A120 A119 A118 A117 A116 A115 A114 A113 A112 A111 A110 A109 A108 A107 A106 A105 A104 A103 A102 A101 A100 A99 A98 A97 A96 A95 A94 A93 A92 A91 A90 A89 A88 A87 A86 A85 A84 A83 A82 A81 A80 A79 A78 A77 A76 A75 A74 A73 A72 A71 A70 A69 A68 A67 A66 A65 A64 A63 A62 A61 A60 A59 A58 A57 | A13 A150 A31 A258 A259 A260 A32 A261 A262 A11 | A11 A279 A47 A48 A49 A12 | A262 A261 A32 A33 A34 A35 A36 A37 A38 A39 A12 A11 | A13 A4 A248 A249 A250 A251 A252 A253 A254 A255 A256 A257 A258 A31 A150 | A11 A286 A285 A284 A43 A44 A283 A282 A281 A280 A47 A279 | A49 A48 A47 A279 A280 A12 | A12 A47 A46 A39 A38 A37 A36 A35 A34 A33 A32 A261 A260 A31 A258 A257 A256 A255 A254 A253 A252 A251 A250 A249 A248 A4 A246 A245 A244 A242 A241 A240 A239 A238 A237 A236 A235 A234 A233 A232 A231 A230 A55 A54 A53 A52 A51 A50 A49 | A56 A55 A228 | A12 A39 A40 A41 A42 A43 A284 A285 A286 A11 A287 A288 A289 | A47 A280 A279 | A47 A280 A281 A282 A283 A44 A45 A46 A12 | A12 A46 A47 | A228 A229 A230 A55 | A244 A245 A246 A4 | A289 A288 A287 A11 | A12 A46 A45 A44 A283 A284 A43 A42 A41 A40 A39 | A32 A31 A260 A261 | A31 A260 A259 A258 | A284 A283 A44 A43 | A2 | L3 L9 L5 L11 L8 L12 L10 L6 A7 L2 L1 L23 L22 L21 L20 L16 L13 L17 L18 L19 L0 | L24 L25 L26 L3 | L3 A5 L9 | L3 A25 L32 A26 L33 L4 L11 L5 A5 | L3 L33 A26 L32 A25 | A7 L6 L10 L7 L2 | L3 L8 L4 | L7 L12 L3 L2 | L27 A15 L28 A16 | L34 A28 L35 A27
extrude "Extrusion6" add sketch "Sketch1" along normal blind 6.2 contours A0 A178 A179 A180 A181 A182 A183 A184 A185 A186 A187 A188 A189 A190 A191 A192 A193 A194 A195 A196 A197 A198 A199 A200 A201 A202 A203 A204 A205 A206 A207 A208 A209 A210 A211 A212 A213 A214 A215 A216 A217 A218 A219 A220 A221 A222 A223 A224 A225 A226 A227 A11 A13 | A13 A11 A262 A263 A264 A265 A266 A267 A268 A269 A270 A271 A152 A153 A154 A155 A156 A157 A158 A159 A0 | A0 A159 A158 A157 A156 A155 A154 A153 A152 A271 A270 A269 A268 A267 A266 A265 A264 A263 A262 A11 A12 A227 A226 A225 A224 A223 A222 A221 A220 A219 A218 A217 A216 A215 A214 A213 A212 A211 A210 A209 A208 A207 A206 A205 A204 A203 A202 A201 A200 A199 A198 A197 A196 A195 A194 A193 A192 A191 A190 A189 A188 A187 A186 A185 A184 A183 A182 A181 A180 A179 A178 | A2 | L3 L9 L5 L11 L8 L12 L10 L6 A7 L2 L1 L23 L22 L21 L20 L16 L13 L17 L18 L19 L0 | L24 L25 L26 L3 | L3 A5 L9 | L3 A25 L32 A26 L33 L4 L11 L5 A5 | L3 L33 A26 L32 A25 | A7 L6 L10 L7 L2 | L3 L8 L4 | L7 L12 L3 L2 | L27 A15 L28 A16 | L34 A28 L35 A27
ref_plane "Work Plane3" through (6.7641, -40.8581, 9.3) normal (0, 0, 1) x (0.9993859, -0.0350396, 0)
extrude "Extrusion7" add sketch "Sketch1" along normal up to surface (9.3 mm away) contours A2 | L3 L9 L5 L11 L8 L12 L10 L6 A7 L2 L1 L23 L22 L21 L20 L16 L13 L17 L18 L19 L0 | L24 L25 L26 L3 | L3 A5 L9 | L3 A25 L32 A26 L33 L4 L11 L5 A5 | L3 L33 A26 L32 A25 | A7 L6 L10 L7 L2 | L3 L8 L4 | L7 L12 L3 L2 | L27 A15 L28 A16 | L34 A28 L35 A27
extrude "Extrusion8" cut sketch "Sketch1" along normal blind 3 contours A2 | L3 A5 L9 | L3 A25 L32 A26 L33 L4 L11 L5 A5 | L3 L33 A26 L32 A25 | A7 L6 L10 L7 L2 | L2 L7 A7 | L3 L8 L4 | L7 L12 L3 L2 | L34 A28 L35 A27
body "Solid2"
